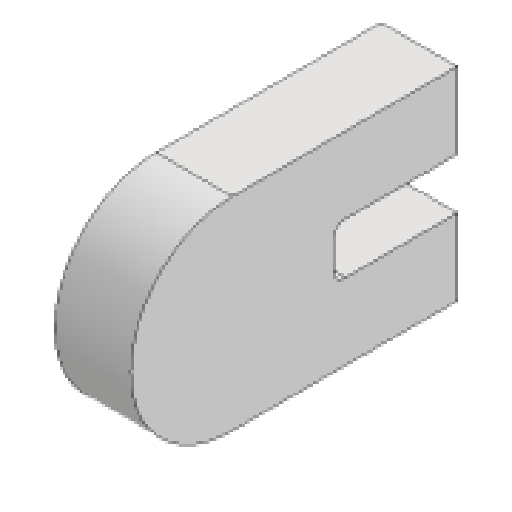
# Autodesk Inventor part: 4barServoSide
Saved by Autodesk Inventor 2023 (Build 270158000, 158)
## iProperties
Created: 2022-10-28
Part Number: 4barServoSide
Material: Generic
Document SubType Name: Modeling
Designer: deli
Density: 1 g/cm^3
Appearance: Default
Author: deli
Autodesk Inventor part; units mm, degrees
ref_plane "YZ Plane" through (0, 0, 0) normal (1, 0, 0) x (0, 1, 0)
ref_plane "XZ Plane" through (0, 0, 0) normal (0, 1, 0) x (-1, 0, 0)
ref_plane "XY Plane" through (0, 0, 0) normal (0, 0, 1) x (1, 0, 0)
sketch "Sketch1" plane through (0, 0, 0) normal (1, 0, 0) x (0, 1, 0)
  circle A0 centre (21.1079, 1.8573) radius 16
  line L0 (37.1079, -33.6346) -> (25.1079, -33.6346)
  line L1 (25.1079, -33.6346) -> (25.1079, -13.6346)
  line L2 (25.1079, -13.6346) -> (37.1079, -13.6346)
  line L3 (37.1079, -13.6346) -> (37.1079, -33.6346)
  line L4 (17.1079, -13.6346) -> (5.1079, -13.6346)
  line L5 (5.1079, -13.6346) -> (5.1079, -33.6346)
  line L6 (5.1079, -33.6346) -> (17.1079, -33.6346)
  line L7 (17.1079, -33.6346) -> (17.1079, -13.6346)
  line L8 (37.1079, -13.6346) -> (37.1079, 1.8573)
  line L9 (5.1079, -13.6346) -> (5.1079, 1.8573)
  point P0 (0, 0)
  dimension "d0" = 32
  dimension "d1" = 12
  dimension "d2" = 20
  constraints: 20 end point, 5 parallel, 4 point on circle, 2 equal length, 2 horizontal, 2 perpendicular, 2 tangent, 1 centre point, 1 vertical
  measures "d0" diameter of A0
  measures "d1" distance of L1.end L2.end
  measures "d2" distance of L0.end L1.end
extrude "Extrusion1" add sketch "Sketch1" along normal blind 12
fillet "Fillet1" radius 2 2 edges at (6, 17.1079, -13.6346) (6, 25.1079, -13.6346)
sketch "Sketch2" plane through (0, 0, 0) normal (-1, 0, 0) x (0, 0, 1)
  arc A0 (1.8573, 5.1079) -> (1.8573, 37.1079) centre (1.8573, 21.1079) ccw projected
  circle A1 centre (1.8573, 21.1079) radius 16
  line L0 (-16.0312, 25.1079) -> (-33.6346, 25.1079) projected
  line L1 (-33.6346, 25.1079) -> (-13.6346, 25.1079)
  line L2 (-13.6346, 25.1079) -> (-13.6346, 17.1079)
  line L3 (-13.6346, 17.1079) -> (-33.6346, 17.1079)
  line L4 (-33.6346, 17.1079) -> (-33.6346, 25.1079)
  line L5 (-33.6346, 17.1079) -> (-16.0312, 17.1079) projected
  point P0 (0, 0)
  point P1 (1.8573, 37.1079)
  constraints: 8 end point, 2 parallel, 1 coincident, 1 collinear, 1 horizontal, 1 perpendicular, 4 other
extrude "Extrusion2" cut sketch "Sketch2" against normal blind 6
fillet "Fillet2" radius 2 2 edges at (3, 37.1079, 1.8573) (3, 5.1079, 1.8573)
sketch "Sketch3" plane through (0, 25.1079, -33.6346) normal (0, 0, -1) x (-1, 0, 0)
  circle A0 centre (-6, 6) radius 4
  circle A1 centre (-5.9819, -13.9428) radius 4
  line L0 (-6, 12) -> (-12, 12) construction
  line L1 (-12, 12) -> (0, 0) construction
  line L2 (-12, 0) -> (0, 11.9535) construction
  line L3 (-11.3657, -8.506) -> (0.6343, -20.6243) construction
  line L4 (0, -7.9012) -> (0, -9.2455) construction
  line L5 (-11.9754, -19.9962) -> (0, -7.9012) construction
  point P0 (0, -25.1079)
  point P1 (0, -7.9506)
  dimension "d9" = 8
  dimension "d10" = 8
  constraints: 8 end point, 2 centre point, 2 point on line, 1 coincident, 1 midpoint
  measures "d9" diameter of A0
  measures "d10" diameter of A1
extrude "Extrusion3" cut sketch "Sketch3" against normal blind 18
sketch "Sketch4" plane through (0, 25.1079, -33.6346) normal (0, 0, -1) x (-1, 0, 0)
  circle A0 centre (-6, 6) radius 6
  circle A1 centre (-6, 6) radius 4 projected
  line L0 (-12, 0) -> (-12, 12) projected
  circle A2 centre (-6, -14) radius 6
  circle A3 centre (-5.9819, -13.9428) radius 4 projected
  line L1 (-12, -20) -> (-12, -8) projected
  circle A4 centre (-6, 6) radius 4 projected
  line L2 (0, 0) -> (0, 12) projected
  line L3 (0, 12) -> (-12, 12) projected
  line L4 (-12, 0) -> (-12, 12) projected
  line L5 (0, 0) -> (-12, 0) projected
  circle A5 centre (-5.9819, -13.9428) radius 4 projected
  line L6 (0, -20) -> (0, -8) projected
  line L7 (0, -8) -> (-12, -8) projected
  line L8 (-12, -20) -> (-12, -8) projected
  line L9 (0, -20) -> (-12, -20) projected
  point P0 (0, -25.1079)
  point P1 (-6, -20)
  point P2 (0, -14)
  point P3 (-12, -14)
  point P4 (-6, -8)
  point P5 (-6, 12)
  point P6 (-12, 6)
  point P7 (0, 6)
  point P8 (-6, 0)
  constraints: 4 tangent, 2 centre point, 1 concentric
extrude "Extrusion4" cut sketch "Sketch4" against normal blind 70 contours L2 L5 A0 | A0 L3 L2 | A0 L0 L3 | L6 L9 A2 | A2 L7 L6 | L9 L1 A2
fillet "Fillet3" radius 6 3 edges at (12, 21.1079, -14.1427) (12, 25.1079, -24.8329) (12, 17.1079, -24.8329)
body "Solid1"
